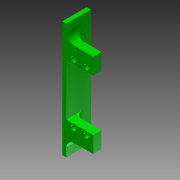
# Autodesk Inventor part: ServoMount
Saved by Autodesk Inventor 2012 (Build 160160000, 160)
## iProperties
Created: 2013-10-06
Part Number: ServoMount
Material: ABS Plastic
Document SubType Name: Modeling
Designer: joe_000
Density: 1.06 g/cm^3
Mass: 3.55612 g
Surface Area: 19.0754 cm^2
Volume: 3.35483 cm^3
ServoMountLength: 3.528 in
Author: joe_000
Autodesk Inventor part; units mm, degrees
ref_plane "YZ Plane" through (0, 0, 0) normal (1, 0, 0) x (0, 1, 0)
ref_plane "XZ Plane" through (0, 0, 0) normal (0, 1, 0) x (-1, 0, 0)
ref_plane "XY Plane" through (0, 0, 0) normal (0, 0, 1) x (1, 0, 0)
sketch "Sketch1" plane through (0, 0, 0) normal (0, 0, 1) x (1, 0, 0)
  line L0 (0, 0) -> (20.8, 0)
  line L1 (20.8, 0) -> (20.8, 12.7)
  line L2 (20.8, 12.7) -> (0, 12.7)
  line L3 (0, 12.7) -> (0, 0)
  line L4 (0, -39.8112) -> (20.8, -39.8112)
  line L5 (20.8, -39.8112) -> (20.8, -52.5112)
  line L6 (20.8, -52.5112) -> (0, -52.5112)
  line L7 (0, -52.5112) -> (0, -39.8112)
  line L8 (10.4, 12.7) -> (10.4, 0)
  point P0 (5.4, 3)
  dimension "d0" = 20.8
  dimension "d1" = 12.7
  dimension "d2" = 39.8112
  dimension "d33" = 3
  dimension "d34" = 5
  dimension "d41" = 10.4
  constraints: 18 end point, 4 parallel, 3 collinear, 3 perpendicular, 2 horizontal, 2 midpoint
  measures "d0" distance of L1.end L2.end
  measures "d1" distance of L0.end L1.end
  measures "d2" distance between parallel lines of L4 L0
  measures "d33" distance from line of L0 point (5.4, 3)
  measures "d34" distance from line of L8 point (5.4, 3)
  measures "d41" distance between parallel lines of L3 L8
extrude "Extrusion1" add sketch "Sketch1" against normal blind 6.35
hole "Hole3" at (5.4, 3, 0) direction (0, 0, -1) diameter 4 depth 25.4
pattern_linear "Rectangular Pattern1" count 2 spacing 10 along (1, 0, 0) count 2 spacing 45.8 along (0, -1, 0) of "Hole3"
sketch "Sketch3" plane through (0, 0, 0) normal (-1, 0, 0) x (0, 0, 1)
  line L0 (0, 12.7) -> (0, 0) projected
  line L1 (-19.05, 24.4) -> (0, 24.4)
  line L2 (0, 24.4) -> (0, -65.2112)
  line L3 (0, -65.2112) -> (-19.05, -65.2112)
  line L4 (-19.05, -65.2112) -> (-19.05, 24.4)
  line L5 (0, -39.8112) -> (-6.35, -39.8112) projected
  dimension "d42" = 19.05
  dimension "ServoMountLength" = 89.6112
  dimension "d45" = 25.4
  constraints: 8 end point, 2 parallel, 1 collinear, 1 horizontal, 1 perpendicular
  measures "d42" distance of L1.start L1.end
  measures "ServoMountLength" distance of L3.end L1.start
  measures "d45" distance between parallel lines of L3 L5
extrude "Extrusion2" add sketch "Sketch3" along normal blind 3.175
fillet "Fillet1" radius 6.35 4 edges at (0, 6.35, -6.35) (0, 12.7, -3.175) (0, -46.1612, -6.35) (0, -52.5112, -3.175)
equation "\"d0\" = ServoWidth + ServoTolerance"
equation "\"d2\" = ServoLength + ServoTolerance"
equation "\"d33\" = ServoScrewOffsetFromSide - 0.5 * ServoTolerance"
equation "\"d34\" = 0.5 * ServoScrewSpacing"
equation "\"d41\" = 0.5 * ServoTolerance + 0.5 * ServoWidth"
equation "\"d37\" = ServoScrewSpacing"
equation "\"d40\" = ServoScrewSpacingLength"
equation "\"ServoTolerance\" = 1"
equation "\"ServoWidth\" = 19.8"
equation "\"ServoLength\" = 38.8112"
equation "\"ServoScrewSpacing\" = 10"
equation "\"ServoScrewSpacingLength\" = 45.8"
equation "\"ServoScrewOffsetFromSide\" = 3.5"
body "Solid1"
